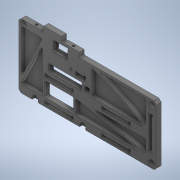
# Autodesk Inventor part: Cockpit_vertical_frame_01
Saved by Autodesk Inventor 2020 (Build 240168000, 168)
## iProperties
Created: 2021-08-10
Part Number: Cockpit_vertical_frame_01
Material: アセタール樹脂、黒
Document SubType Name: Modeling
Designer: Masato
Density: 1.425 g/cm^3
Appearance: 滑らか - 黒
Mass: 38.105 g
Surface Area: 250.223 cm^2
Volume: 26.7404 cm^3
d0: 145.000 mm
d3: 81.000 mm
d4: 0.050 mm
d6: 2.100 mm
d7: 0.050 mm
d8: 0.050 mm
d9: 13.800 mm
d10: 9.200 mm
d11: 63.000 mm
d12: 5.000 mm
d15: 2.500 mm
d16: 5.000 mm
d17: 5.000 mm
d19: 30.500 mm
d21: 3.200 mm
d22: 6.000 mm
d23: 2.500 mm
d24: 5.000 mm
d25: 6.000 mm
d26: 3.200 mm
d27: 5.000 mm
d28: 2.500 mm
d29: 2.500 mm
d30: 5.000 mm
d31: 6.000 mm
d32: 3.200 mm
d33: 30.000 mm
d34: 2.500 mm
d35: 1.050 mm
d37: 0.050 mm
d38: 0.050 mm
d45: 30.000 mm
d46: 2.500 mm
d47: 1.050 mm
d48: 0.050 mm
d49: 0.050 mm
d50: 10.500 mm
d51: 2.500 mm
d52: 1.050 mm
d53: 0.050 mm
d54: 0.050 mm
d55: 20.000 mm
d56: 10.000 mm
d57: 10.000 mm
d58: 2.500 mm
d59: 30.000 mm
d60: 30.000 mm
d68: 5.000 mm
d69: 5.000 mm
d70: 70.500 mm
d71: 8.000 mm
d72: 12.000 mm
d73: 5.275 mm
d75: 35.000 mm
d76: 60.535 mm
d77: 30.000 mm
d78: 2.500 mm
d79: 1.050 mm
d80: 0.050 mm
d81: 0.050 mm
d82: 30.000 mm
d83: 2.500 mm
d84: 1.050 mm
d85: 0.050 mm
d86: 0.050 mm
d87: 1.050 mm
d88: 1.050 mm
d89: 26.333 mm
d90: 18.833 mm
d91: 5.000 mm
d104: 20.000 mm
d105: 8.000 mm
d106: 2.100 mm
d107: 0.050 mm
d108: 0.050 mm
d109: 15.100 mm
d110: 10.600 mm
d111: 23.500 mm
d112: 5.000 mm
d113: 9.000 mm
d114: 2.500 mm
d115: 4.000 mm
d116: 15.000 mm
d121: 5.000 mm
d122: 0.00 deg
d123: 2.000 mm
d124: 0.00 deg
d125: 0.050 mm
d126: 0.050 mm
d127: 1.050 mm
d128: 2.500 mm
d129: 35.000 mm
d130: 2.500 mm
d133: 1.000 mm
d137: 4.000 mm
d141: 4.000 mm
d142: 118.00 deg
d147: 6.000 mm
d148: 3.200 mm
d149: 6.000 mm
d150: 3.200 mm
d151: 6.000 mm
d152: 3.200 mm
d153: 6.000 mm
d154: 3.200 mm
Author: Masato
Autodesk Inventor part; units mm, degrees
ref_plane "YZ Plane" through (0, 0, 0) normal (1, 0, 0) x (0, 1, 0)
ref_plane "XZ Plane" through (0, 0, 0) normal (0, 1, 0) x (-1, 0, 0)
ref_plane "XY Plane" through (0, 0, 0) normal (0, 0, 1) x (1, 0, 0)
sketch "スケッチ1" plane through (0, 0, 0) normal (0, 0, 1) x (1, 0, 0)
  line L0 (0, 0) -> (145, 0)
  line L1 (145, 0) -> (145, 63)
  line L2 (64, 68) -> (64, 63)
  line L3 (0, 68) -> (0, 0)
  line L4 (37.05, 64.65) -> (38.5349, 64.65) construction
  line L5 (50.95, 64.65) -> (50.95, 63.1651) construction
  line L6 (50.95, 55.35) -> (49.4651, 55.35) construction
  line L7 (37.05, 55.35) -> (37.05, 56.8349) construction
  line L8 (37.05, 64.65) -> (50.95, 55.35) construction
  line L9 (50.95, 64.65) -> (37.05, 55.35) construction
  line L10 (37.1, 64.6) -> (50.9, 64.6) construction
  line L11 (50.9, 64.6) -> (50.9, 55.4) construction
  line L12 (50.9, 55.4) -> (37.1, 55.4) construction
  line L13 (37.1, 55.4) -> (37.1, 64.6) construction
  line L14 (37.1, 64.6) -> (50.9, 55.4) construction
  line L15 (50.9, 64.6) -> (37.1, 55.4) construction
  arc A0 (38.5349, 64.65) -> (37.05, 63.1651) centre (37.7925, 63.9075) ccw
  line L16 (38.5349, 64.65) -> (37.05, 63.1651) construction
  line L17 (37.7925, 63.9075) -> (37.05, 64.65) construction
  line L18 (37.05, 60) -> (50.95, 60) construction
  line L19 (44, 64.65) -> (44, 55.35) construction
  arc A1 (50.95, 63.1651) -> (49.4651, 64.65) centre (50.2075, 63.9075) ccw
  arc A2 (37.05, 56.8349) -> (38.5349, 55.35) centre (37.7925, 56.0925) ccw
  arc A3 (49.4651, 55.35) -> (50.95, 56.8349) centre (50.2075, 56.0925) ccw
  line L20 (38.5349, 64.65) -> (49.4651, 64.65)
  line L21 (37.05, 63.1651) -> (37.05, 64.65) construction
  line L22 (49.4651, 64.65) -> (50.95, 64.65) construction
  line L23 (50.95, 63.1651) -> (50.95, 56.8349)
  line L24 (37.05, 56.8349) -> (37.05, 63.1651)
  line L25 (38.5349, 55.35) -> (37.05, 55.35) construction
  line L26 (49.4651, 55.35) -> (38.5349, 55.35)
  line L27 (50.95, 56.8349) -> (50.95, 55.35) construction
  line L28 (64, 63) -> (145, 63)
  line L29 (27.5, 23.9) -> (57.5, 23.9)
  line L30 (57.5, 23.9) -> (57.5, 8.6)
  line L31 (57.5, 8.6) -> (27.5, 8.6)
  line L32 (27.5, 8.6) -> (27.5, 23.9)
  line L33 (27.5, 23.9) -> (57.5, 8.6) construction
  line L34 (57.5, 23.9) -> (27.5, 8.6) construction
  line L35 (137.5, 63) -> (137.5, 0) construction
  line L36 (142.5, 63) -> (142.5, 0) construction
  line L37 (0, 32.5) -> (137.5, 32.5) construction
  line L38 (137.5, 27.5) -> (0, 27.5) construction
  line L39 (137.5, 31.5) -> (142.5, 31.5) construction
  circle A4 centre (140, 5) radius 1.6
  circle A5 centre (140, 5) radius 3
  circle A6 centre (140, 58) radius 1.6
  circle A7 centre (140, 58) radius 3
  arc A8 (19.1583, 0) -> (15.8417, 0) centre (17.5, 2.5) ccw
  circle A9 centre (17.5, 2.5) radius 1.6
  line L40 (2.5, 27.5) -> (2.5, 0) construction
  line L41 (7.5, 0) -> (7.5, 27.5) construction
  line L42 (7.5, 5) -> (137.5, 5) construction
  arc A10 (69.1583, 0) -> (65.8417, 0) centre (67.5, 2.5) ccw
  circle A11 centre (67.5, 2.5) radius 1.6
  line L43 (27.5, 5) -> (57.5, 5) construction
  line L44 (57.5, 5) -> (57.5, 2.5) construction
  line L45 (57.5, 2.5) -> (27.5, 2.5) construction
  line L46 (27.5, 2.5) -> (27.5, 5) construction
  line L47 (27.5, 5) -> (57.5, 2.5) construction
  line L48 (57.5, 5) -> (27.5, 2.5) construction
  line L49 (27.45, 5.05) -> (29.55, 5.05) construction
  line L50 (57.55, 5.05) -> (57.55, 2.45)
  line L51 (57.55, 2.45) -> (55.45, 2.45) construction
  line L52 (27.45, 2.45) -> (27.45, 5.05)
  line L53 (27.45, 5.05) -> (57.55, 2.45) construction
  line L54 (57.55, 5.05) -> (27.45, 2.45) construction
  line L55 (27.45, 3.75) -> (57.55, 3.75) construction
  line L56 (42.5, 5.05) -> (42.5, 2.45) construction
  arc A12 (29.55, 5.05) -> (27.45, 5.05) centre (28.5, 5.05) ccw
  arc A13 (27.45, 2.45) -> (29.55, 2.45) centre (28.5, 2.45) ccw
  arc A14 (57.55, 5.05) -> (55.45, 5.05) centre (56.5, 5.05) ccw
  arc A15 (55.45, 2.45) -> (57.55, 2.45) centre (56.5, 2.45) ccw
  line L57 (29.55, 5.05) -> (55.45, 5.05)
  line L58 (29.55, 2.45) -> (27.45, 2.45) construction
  line L59 (55.45, 5.05) -> (57.55, 5.05) construction
  line L60 (55.45, 2.45) -> (29.55, 2.45)
  line L61 (87.5, 5) -> (117.5, 5) construction
  line L62 (117.5, 5) -> (117.5, 2.5) construction
  line L63 (117.5, 2.5) -> (87.5, 2.5) construction
  line L64 (87.5, 2.5) -> (87.5, 5) construction
  line L65 (87.5, 5) -> (117.5, 2.5) construction
  line L66 (117.5, 5) -> (87.5, 2.5) construction
  line L67 (87.45, 5.05) -> (89.55, 5.05) construction
  line L68 (117.55, 5.05) -> (117.55, 2.45)
  line L69 (117.55, 2.45) -> (115.45, 2.45) construction
  line L70 (87.45, 2.45) -> (87.45, 5.05)
  line L71 (87.45, 5.05) -> (117.55, 2.45) construction
  line L72 (117.55, 5.05) -> (87.45, 2.45) construction
  line L73 (87.45, 3.75) -> (117.55, 3.75) construction
  line L74 (102.5, 5.05) -> (102.5, 2.45) construction
  arc A16 (89.55, 5.05) -> (87.45, 5.05) centre (88.5, 5.05) ccw
  arc A17 (87.45, 2.45) -> (89.55, 2.45) centre (88.5, 2.45) ccw
  arc A18 (117.55, 5.05) -> (115.45, 5.05) centre (116.5, 5.05) ccw
  arc A19 (115.45, 2.45) -> (117.55, 2.45) centre (116.5, 2.45) ccw
  line L75 (89.55, 5.05) -> (115.45, 5.05)
  line L76 (89.55, 2.45) -> (87.45, 2.45) construction
  line L77 (115.45, 5.05) -> (117.55, 5.05) construction
  line L78 (115.45, 2.45) -> (89.55, 2.45)
  line L79 (68.45, 48.05) -> (70.55, 48.05) construction
  line L80 (60, 48) -> (70.5, 48) construction
  line L81 (70.5, 48) -> (70.5, 45.5) construction
  line L82 (65.25, 48.05) -> (65.25, 45.45) construction
  line L83 (62.05, 48.05) -> (68.45, 48.05)
  line L84 (68.45, 45.45) -> (62.05, 45.45)
  line L85 (70.5, 45.5) -> (60, 45.5) construction
  line L86 (60, 48) -> (70.5, 45.5) construction
  line L87 (59.95, 48.05) -> (70.55, 45.45) construction
  line L88 (70.55, 48.05) -> (59.95, 45.45) construction
  line L89 (59.95, 46.75) -> (70.55, 46.75) construction
  line L90 (70.5, 48) -> (60, 45.5) construction
  arc A20 (68.45, 45.45) -> (70.55, 45.45) centre (69.5, 45.45) ccw
  line L91 (70.55, 45.45) -> (68.45, 45.45) construction
  line L92 (70.55, 48.05) -> (70.55, 45.45)
  arc A21 (70.55, 48.05) -> (68.45, 48.05) centre (69.5, 48.05) ccw
  arc A22 (62.05, 48.05) -> (59.95, 48.05) centre (61, 48.05) ccw
  line L93 (60, 45.5) -> (60, 48) construction
  line L94 (59.95, 48.05) -> (62.05, 48.05) construction
  line L95 (59.95, 45.45) -> (59.95, 48.05)
  line L96 (62.05, 45.45) -> (59.95, 45.45) construction
  arc A23 (59.95, 45.45) -> (62.05, 45.45) centre (61, 45.45) ccw
  line L97 (69.5, 40.275) -> (74.5, 40.275)
  line L98 (74.5, 40.275) -> (74.5, 35.275)
  line L99 (74.5, 35.275) -> (69.5, 35.275)
  line L100 (69.5, 35.275) -> (69.5, 40.275)
  line L101 (69.5, 40.275) -> (74.5, 35.275) construction
  line L102 (74.5, 40.275) -> (69.5, 35.275) construction
  line L103 (54.535, 41.775) -> (66.535, 41.775)
  line L104 (66.535, 41.775) -> (66.535, 33.775)
  line L105 (66.535, 33.775) -> (54.535, 33.775)
  line L106 (54.535, 33.775) -> (54.535, 41.775) construction
  line L107 (54.535, 41.775) -> (66.535, 33.775) construction
  line L108 (66.535, 41.775) -> (54.535, 33.775) construction
  line L109 (31.535, 33.775) -> (31.535, 41.775)
  line L110 (31.535, 41.775) -> (54.535, 41.775)
  line L111 (54.535, 33.775) -> (31.535, 33.775)
  line L112 (54.535, 37.775) -> (66.535, 37.775) construction
  line L113 (55.45, 30.05) -> (57.55, 30.05) construction
  arc A24 (57.55, 30.05) -> (55.45, 30.05) centre (56.5, 30.05) ccw
  line L114 (57.5, 30) -> (57.5, 27.5) construction
  line L115 (57.55, 30.05) -> (57.55, 27.45)
  arc A25 (55.45, 27.45) -> (57.55, 27.45) centre (56.5, 27.45) ccw
  line L116 (57.55, 27.45) -> (55.45, 27.45) construction
  line L117 (27.5, 30) -> (57.5, 30) construction
  line L118 (42.5, 30.05) -> (42.5, 27.45) construction
  line L119 (29.55, 30.05) -> (55.45, 30.05)
  line L120 (55.45, 27.45) -> (29.55, 27.45)
  line L121 (27.45, 28.75) -> (57.55, 28.75) construction
  line L122 (27.45, 30.05) -> (57.55, 27.45) construction
  line L123 (57.55, 30.05) -> (27.45, 27.45) construction
  line L124 (57.5, 27.5) -> (27.5, 27.5) construction
  line L125 (27.5, 30) -> (57.5, 27.5) construction
  line L126 (57.5, 30) -> (27.5, 27.5) construction
  arc A26 (27.45, 27.45) -> (29.55, 27.45) centre (28.5, 27.45) ccw
  line L127 (29.55, 27.45) -> (27.45, 27.45) construction
  line L128 (27.5, 27.5) -> (27.5, 30) construction
  line L129 (27.45, 27.45) -> (27.45, 30.05)
  line L130 (27.45, 30.05) -> (29.55, 30.05) construction
  arc A27 (29.55, 30.05) -> (27.45, 30.05) centre (28.5, 30.05) ccw
  line L131 (115.45, 30.05) -> (117.55, 30.05) construction
  arc A28 (117.55, 30.05) -> (115.45, 30.05) centre (116.5, 30.05) ccw
  line L132 (117.5, 30) -> (117.5, 27.5) construction
  line L133 (117.55, 30.05) -> (117.55, 27.45)
  arc A29 (115.45, 27.45) -> (117.55, 27.45) centre (116.5, 27.45) ccw
  line L134 (117.55, 27.45) -> (115.45, 27.45) construction
  line L135 (87.5, 30) -> (117.5, 30) construction
  line L136 (102.5, 30.05) -> (102.5, 27.45) construction
  line L137 (89.55, 30.05) -> (115.45, 30.05)
  line L138 (115.45, 27.45) -> (89.55, 27.45)
  line L139 (87.45, 28.75) -> (117.55, 28.75) construction
  line L140 (87.45, 30.05) -> (117.55, 27.45) construction
  line L141 (117.55, 30.05) -> (87.45, 27.45) construction
  line L142 (117.5, 27.5) -> (87.5, 27.5) construction
  line L143 (87.5, 30) -> (117.5, 27.5) construction
  line L144 (117.5, 30) -> (87.5, 27.5) construction
  arc A30 (87.45, 27.45) -> (89.55, 27.45) centre (88.5, 27.45) ccw
  line L145 (89.55, 27.45) -> (87.45, 27.45) construction
  line L146 (87.5, 27.5) -> (87.5, 30) construction
  line L147 (87.45, 27.45) -> (87.45, 30.05)
  line L148 (87.45, 30.05) -> (89.55, 30.05) construction
  arc A31 (89.55, 30.05) -> (87.45, 30.05) centre (88.5, 30.05) ccw
  line L149 (26.3333, 73) -> (45.1667, 73)
  line L150 (26.3333, 73) -> (26.3333, 68)
  arc A32 (24.2333, 68) -> (26.3333, 68) centre (25.2833, 68) ccw
  line L151 (0, 68) -> (24.2333, 68)
  line L152 (45.1667, 73) -> (45.1667, 68)
  line L153 (47.2667, 68) -> (64, 68)
  arc A33 (45.1667, 68) -> (47.2667, 68) centre (46.2167, 68) ccw
  line L154 (36.4, 65.35) -> (37.8849, 65.35) construction
  line L155 (51.6, 65.35) -> (51.6, 63.8651) construction
  line L156 (51.6, 54.65) -> (50.1151, 54.65) construction
  line L157 (36.4, 54.65) -> (36.4, 56.1349) construction
  line L158 (36.4, 65.35) -> (51.6, 54.65) construction
  line L159 (51.6, 65.35) -> (36.4, 54.65) construction
  line L160 (36.45, 65.3) -> (51.55, 65.3) construction
  line L161 (51.55, 65.3) -> (51.55, 54.7) construction
  line L162 (51.55, 54.7) -> (36.45, 54.7) construction
  line L163 (36.45, 54.7) -> (36.45, 65.3) construction
  line L164 (36.45, 65.3) -> (51.55, 54.7) construction
  line L165 (51.55, 65.3) -> (36.45, 54.7) construction
  arc A34 (37.8849, 65.35) -> (36.4, 63.8651) centre (37.1425, 64.6075) ccw
  line L166 (37.8849, 65.35) -> (36.4, 63.8651) construction
  line L167 (37.1425, 64.6075) -> (36.4, 65.35) construction
  line L168 (36.4, 60) -> (51.6, 60) construction
  line L169 (44, 65.35) -> (44, 54.65) construction
  arc A35 (51.6, 63.8651) -> (50.1151, 65.35) centre (50.8575, 64.6075) ccw
  arc A36 (36.4, 56.1349) -> (37.8849, 54.65) centre (37.1425, 55.3925) ccw
  arc A37 (50.1151, 54.65) -> (51.6, 56.1349) centre (50.8575, 55.3925) ccw
  line L170 (37.8849, 65.35) -> (50.1151, 65.35)
  line L171 (36.4, 63.8651) -> (36.4, 65.35) construction
  line L172 (50.1151, 65.35) -> (51.6, 65.35) construction
  line L173 (51.6, 63.8651) -> (51.6, 56.1349)
  line L174 (36.4, 56.1349) -> (36.4, 63.8651)
  line L175 (37.8849, 54.65) -> (36.4, 54.65) construction
  line L176 (50.1151, 54.65) -> (37.8849, 54.65)
  line L177 (51.6, 56.1349) -> (51.6, 54.65) construction
  line L178 (51, 50.5) -> (74.5, 50.5) construction
  line L179 (74.5, 50.5) -> (74.5, 45.5) construction
  line L180 (74.5, 45.5) -> (51, 45.5) construction
  line L181 (51, 45.5) -> (51, 50.5) construction
  line L182 (51, 48) -> (74.5, 48) construction
  circle A38 centre (55, 48) radius 1.25
  line L183 (137.45, 49.05) -> (140.05, 49.05)
  line L184 (140.05, 49.05) -> (140.05, 46.95)
  line L185 (140.05, 13.95) -> (137.45, 13.95)
  line L186 (137.45, 13.95) -> (137.45, 16.05) construction
  line L187 (137.45, 49.05) -> (140.05, 13.95) construction
  line L188 (140.05, 49.05) -> (137.45, 13.95) construction
  line L189 (137.5, 49) -> (140, 49) construction
  line L190 (140, 49) -> (140, 14) construction
  line L191 (140, 14) -> (137.5, 14) construction
  line L192 (137.5, 14) -> (137.5, 49) construction
  line L193 (137.5, 49) -> (140, 14) construction
  line L194 (140, 49) -> (137.5, 14) construction
  line L195 (137.45, 31.5) -> (140.05, 31.5) construction
  line L196 (138.75, 49.05) -> (138.75, 13.95) construction
  arc A39 (137.45, 49.05) -> (137.45, 46.95) centre (137.45, 48) ccw
  arc A40 (140.05, 46.95) -> (140.05, 49.05) centre (140.05, 48) ccw
  arc A41 (137.45, 16.05) -> (137.45, 13.95) centre (137.45, 15) ccw
  arc A42 (140.05, 13.95) -> (140.05, 16.05) centre (140.05, 15) ccw
  line L197 (137.45, 46.95) -> (137.45, 49.05) construction
  line L198 (140.05, 46.95) -> (140.05, 16.05)
  line L199 (137.45, 16.05) -> (137.45, 46.95)
  line L200 (140.05, 16.05) -> (140.05, 13.95) construction
  line L201 (3.4, 68) -> (55.9646, 68) construction
  circle A43 centre (5, 64.5) radius 3
  circle A44 centre (5, 64.5) radius 1.6
  line L202 (7.5, 68) -> (7.5, 60.5) construction
  line L203 (7.5, 60.5) -> (2.5, 60.5) construction
  line L204 (2.5, 60.5) -> (2.5, 68) construction
  line L205 (60, 23.9) -> (60, 8.6)
  line L206 (72.3312, 23.9) -> (75.3, 23.9) construction
  line L207 (60, 8.6) -> (133.9, 8.6)
  line L208 (133.9, 11.153) -> (133.9, 23.9)
  line L209 (133.9, 23.9) -> (72.3312, 23.9)
  line L210 (60, 23.9) -> (133.9, 8.6)
  line L211 (72.3312, 23.9) -> (133.9, 11.153)
  line L212 (77, 60.5) -> (77, 33.6)
  line L213 (77, 33.6) -> (133.9, 33.6)
  line L214 (133.9, 36.3653) -> (133.9, 60.5)
  line L215 (133.9, 60.5) -> (82.8493, 60.5)
  line L216 (77, 60.5) -> (133.9, 33.6)
  line L217 (82.8493, 60.5) -> (133.9, 36.3653)
  line L218 (2.5, 61) -> (25, 61)
  line L219 (25, 61) -> (2.5, 14.3543)
  line L220 (2.5, 14.3543) -> (2.5, 61)
  line L221 (25, 55.2457) -> (2.5, 8.6)
  line L222 (2.5, 8.6) -> (25, 8.6)
  line L223 (25, 8.6) -> (25, 55.2457)
  point P0 (44, 60)
  point P1 (44, 60)
  point P2 (42.5, 16.25)
  point P3 (42.5, 3.75)
  point P4 (102.5, 3.75)
  point P5 (65.25, 46.75)
  point P6 (42.5, 16.25)
  point P7 (72, 37.775)
  point P8 (60.535, 37.775)
  point P9 (72, 37.775)
  point P10 (42.5, 28.75)
  point P11 (102.5, 28.75)
  point P12 (44, 60)
  point P13 (44, 60)
  point P14 (138.75, 31.5)
  point P15 (138.75, 31.5)
  dimension "d0" = 145
  dimension "d3" = 81
  dimension "d6" = 2.1
  dimension "d7" = 0.05
  dimension "d8" = 0.05
  dimension "d9" = 13.8
  dimension "d10" = 9.2
  dimension "d11" = 63
  dimension "d12" = 5
  dimension "d15" = 2.5
  dimension "d16" = 5
  dimension "d17" = 5
  dimension "d19" = 30.5
  dimension "d21" = 3.2
  dimension "d22" = 6
  dimension "d23" = 2.5
  dimension "d24" = 5
  dimension "d25" = 6
  dimension "d26" = 3.2
  dimension "d27" = 5
  dimension "d28" = 2.5
  dimension "d29" = 2.5
  dimension "d30" = 5
  dimension "d31" = 6
  dimension "d32" = 3.2
  dimension "d33" = 30
  dimension "d34" = 2.5
  dimension "d35" = 1.05
  dimension "d37" = 0.05
  dimension "d38" = 0.05
  dimension "d45" = 30
  dimension "d46" = 2.5
  dimension "d47" = 1.05
  dimension "d48" = 0.05
  dimension "d49" = 0.05
  dimension "d50" = 10.5
  dimension "d51" = 2.5
  dimension "d52" = 1.05
  dimension "d53" = 0.05
  dimension "d54" = 0.05
  dimension "d55" = 20
  dimension "d56" = 10
  dimension "d57" = 10
  dimension "d58" = 2.5
  dimension "d59" = 30
  dimension "d60" = 30
  dimension "d68" = 5
  dimension "d69" = 5
  dimension "d70" = 70.5
  dimension "d71" = 8
  dimension "d72" = 12
  dimension "d73" = 5.275
  dimension "d75" = 35
  dimension "d76" = 60.535
  dimension "d77" = 30
  dimension "d78" = 2.5
  dimension "d79" = 1.05
  dimension "d80" = 0.05
  dimension "d81" = 0.05
  dimension "d82" = 30
  dimension "d83" = 2.5
  dimension "d84" = 1.05
  dimension "d85" = 0.05
  dimension "d86" = 0.05
  constraints: 446 end point, 124 parallel, 89 midpoint, 74 point on circle, 66 perpendicular, 56 symmetric about line, 45 centre point, 43 horizontal, 28 point on line, 15 collinear, 9 vertical, 7 coincident, 37 other
  measures "d0" distance of L1.start L3.end
  measures "d3" distance of L1.end L2.end
  measures "d6" diameter of A0
  measures "d7" distance from line of L19.start L10
  measures "d8" distance from line of L18.start L13
  measures "d9" distance of L10.end L10.start
  measures "d10" distance of L10.start L12.end
  measures "d11" distance of L1.start L1.end
  measures "d12" distance of L2.end L2.start
  measures "d15" distance of L1.start L36.end
  measures "d16" distance of L35.end L36.end
  measures "d17" distance of L38.end L37.start
  measures "d19" distance of L37.end L35.start
  measures "d21" diameter of A4
  measures "d22" diameter of A5
  measures "d23" horizontal distance of A4.centre L36.end
  measures "d24" vertical distance of L36.end A4.centre
  measures "d25" diameter of A8
  measures "d26" diameter of A9
  measures "d27" distance of L35.end L42.end
  measures "d28" vertical distance of L41.start A8.centre
  measures "d29" distance of L40.end L3.end
  measures "d30" distance of L41.start L40.end
  measures "d31" diameter of A10
  measures "d32" diameter of A11
  measures "d33" distance of L44.end L45.end
  measures "d34" distance of L43.end L44.end
  measures "d35" radius of A12
  measures "d37" distance from line of L46 L55.start
  measures "d38" distance from line of L43 L56.start
  measures "d45" distance of L62.end L63.end
  measures "d46" distance of L61.end L62.end
  measures "d47" radius of A16
  measures "d48" distance from line of L64 L73.start
  measures "d49" distance from line of L61 L74.start
  measures "d50" distance of L81.end L85.end
  measures "d51" distance of L81.start L81.end
  measures "d52" radius of A22
  measures "d53" distance from line of L93 L89.start
  measures "d54" distance from line of L80 L82.start
  measures "d55" distance from line of L46 L42.start
  measures "d56" distance from line of L46 A8.centre
  measures "d57" distance from line of A10.centre L44
  measures "d58" vertical distance of L41.start A10.centre
  measures "d59" distance of L29.end L29.start
  measures "d60" distance between parallel lines of L64 L44
  measures "d68" distance of L98.end L99.end
  measures "d69" distance of L97.end L98.end
  measures "d70" horizontal distance of L1.end L97.end
  measures "d71" distance of L104.end L103.end
  measures "d72" distance of L103.end L103.start
  measures "d73" distance from line of L37 point (60.535, 37.775)
  measures "d75" distance of L103.end L109.end
  measures "d76" horizontal distance of L3.start point (60.535, 37.775)
  measures "d77" distance of L114.end L126.end
  measures "d78" distance of L114.start L114.end
  measures "d79" radius of A27
  measures "d80" distance from line of L128 L121.start
  measures "d81" distance from line of L117 L118.start
  measures "d82" distance of L132.end L144.end
  measures "d83" distance of L132.start L132.end
  measures "d84" radius of A31
  measures "d85" distance from line of L146 L139.start
  measures "d86" distance from line of L135 L136.start
extrude "押し出し1" add sketch "スケッチ1" along normal blind 5 contours L3 L151 A32 L150 L149 L152 A33 L153 L2 L28 L1 L0 A10 A8
extrude "押し出し2" add sketch "スケッチ1" along normal blind 2 contours A8 L0 | A10 L0 | A5 | A7 | L170 A35 L173 A37 L176 A36 L174 A34 | A43
chamfer "面取り1" distance 2.5 angle 45 4 edges at (145, 63, 2.5) (145, 0, 2.5) (0, 0, 2.5) (0, 68, 2.5)
fillet "フィレット1" radius 1 35 edges at (15.8417, 0, 3.5) (19.1583, 0, 3.5) (65.8417, 0, 3.5) (69.1583, 0, 3.5) (31.535, 41.775, 2.5) (31.535, 33.775, 2.5) (66.535, 41.775, 2.5) (66.535, 33.775, 2.5) (69.5, 40.275, 2.5) (69.5, 35.275, 2.5) (74.5, 40.275, 2.5) (74.5, 35.275, 2.5) (27.5, 23.9, 2.5) (27.5, 8.6, 2.5) (57.5, 8.6, 2.5) (57.5, 23.9, 2.5) (64, 63, 2.5) (60, 23.9, 2.5) (60, 8.6, 2.5) (133.9, 8.6, 2.5) (133.9, 11.153, 2.5) (133.9, 23.9, 2.5) (72.3312, 23.9, 2.5) (77, 60.5, 2.5) (77, 33.6, 2.5) (133.9, 33.6, 2.5) (133.9, 36.3653, 2.5) (82.8493, 60.5, 2.5) (133.9, 60.5, 2.5) (2.5, 14.3543, 2.5) (2.5, 8.6, 2.5) (25, 8.6, 2.5) (25, 55.2457, 2.5) (25, 61, 2.5) (2.5, 61, 2.5)
sketch "スケッチ2" plane through (0, 68, 0) normal (0, 1, 0) x (1, 0, 0)
  line L0 (0, 0) -> (0, -5) construction
  line L1 (64, 0) -> (64, -5) construction
  line L2 (24.2333, 0) -> (24.2333, -5) projected
  line L3 (24.2333, -2.5) -> (47.2667, -2.5) construction
  line L4 (47.2667, 0) -> (47.2667, -5) projected
  line L5 (45.1667, 0) -> (45.1667, -5) projected
  line L6 (26.3333, 0) -> (26.3333, -5) projected
  point P0 (16.3333, -2.5)
  point P1 (55.1667, -2.5)
  dimension "d143" = 10
  dimension "d144" = 10
  constraints: 2 end point, 2 midpoint, 2 point on line
  measures "d143" distance from line of L5 point (55.167, -2.5)
  measures "d144" distance from line of L6 point (16.333, -2.5)
hole "穴1" at (16.3333, 68, 2.5) at (55.1667, 68, 2.5) direction (0, -1, 0) diameter 2.459 depth 4 tip angle 118 thread size "M3x0.5" class "6H" standard "ANSI Metric M Profile"
extrude "押し出し3" add sketch "スケッチ1" along normal blind 1 contours L210 L207 L205 | L211 L209 L208 | L216 L213 L212 | L217 L215 L214 | L218 L219 L220 | L223 L222 L221
equation "\"d7\" = d8"
equation "\"d23\" = 0.5 * d16"
equation "\"d25\" = d31"
equation "\"d26\" = d32"
equation "\"d28\" = 0.5 * d27"
equation "\"d31\" = d22"
equation "\"d32\" = d21"
equation "\"d38\" = d37"
